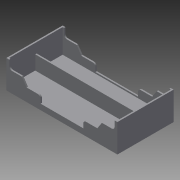
# Autodesk Inventor part: Badrepack
Saved by Autodesk Inventor 2015 (Build 190159000, 159)
## iProperties
Created: 2019-01-15
Part Number: Badrepack
Material: Типовые
Document SubType Name: Modeling
Designer: kostya
Density: 1 g/cm^3
Appearance: По умолчанию
Author: kostya
Autodesk Inventor part; units mm, degrees
ref_plane "YZ Plane" through (0, 0, 0) normal (1, 0, 0) x (0, 1, 0)
ref_plane "XZ Plane" through (0, 0, 0) normal (0, 1, 0) x (-1, 0, 0)
ref_plane "XY Plane" through (0, 0, 0) normal (0, 0, 1) x (1, 0, 0)
sketch "Эскиз1" plane through (0, 0, 0) normal (0, 0, 1) x (1, 0, 0)
  line L0 (-39.5, -20) -> (39.5, -20)
  line L1 (39.5, -20) -> (39.5, 20)
  line L2 (39.5, 20) -> (-39.5, 20)
  line L3 (-39.5, 20) -> (-39.5, -20)
  line L4 (-39.5, -20) -> (39.5, 20) construction
  line L5 (39.5, -20) -> (-39.5, 20) construction
  line L6 (-38.5, 19) -> (38.5, 19)
  line L7 (38.5, 19) -> (38.5, -19)
  line L8 (38.5, -19) -> (-38.5, -19)
  line L9 (-38.5, -19) -> (-38.5, 19)
  point P0 (0, 0)
  dimension "d0" = 79
  dimension "d1" = 40
  dimension "d2" = 1
  constraints: 20 end point, 4 parallel, 2 midpoint, 2 perpendicular, 1 horizontal, 3 other
  measures "d0" distance of L2.end L1.end
  measures "d1" distance of L1.end L0.end
  measures "d2" distance between parallel lines of L2 L6
extrude "Выдавливание1" add sketch "Эскиз1" along normal blind 3 contours L6 L7 L8 L9
extrude "Выдавливание2" add sketch "Эскиз1" along normal blind 20
sketch "Эскиз2" plane through (-39.5, -20, 0) normal (0, -1, 0) x (1, 0, 0)
  line L0 (2, 20) -> (2, 16) construction
  line L1 (4, 14) -> (11, 14)
  arc A0 (2, 16) -> (4, 14) centre (4, 16) ccw
  line L2 (11, 14) -> (11, 9) construction
  line L3 (14.3166, 9) -> (22.3166, 9)
  line L4 (24.3166, 7) -> (24.3166, 4)
  arc A1 (24.3166, 7) -> (22.3166, 9) centre (22.3166, 7) ccw
  line L5 (24.3166, 4) -> (39.5, 4)
  line L6 (39.5, 0) -> (39.5, 20) construction
  line L7 (77, 20) -> (77, 16) construction
  line L8 (75, 14) -> (68, 14)
  arc A2 (75, 14) -> (77, 16) centre (75, 16) ccw
  line L9 (68, 14) -> (64.6834, 9)
  line L10 (64.6834, 9) -> (56.6834, 9)
  line L11 (54.6834, 7) -> (54.6834, 4)
  arc A3 (56.6834, 9) -> (54.6834, 7) centre (56.6834, 7) ccw
  line L12 (54.6834, 4) -> (39.5, 4)
  line L13 (77, 20) -> (77, 16) construction
  line L14 (77, 20) -> (77, 16)
  line L15 (2, 20) -> (77, 20)
  line L16 (14.3166, 9) -> (22.3166, 9)
  line L17 (24.3166, 7) -> (24.3166, 4)
  line L18 (24.3166, 4) -> (54.6834, 4)
  line L19 (54.6834, 4) -> (54.6834, 7)
  line L20 (56.6834, 9) -> (64.6834, 9)
  line L21 (64.6834, 9) -> (68, 14)
  line L22 (68, 14) -> (75, 14)
  line L23 (77, 16) -> (77, 20)
  line L24 (77, 20) -> (2, 20)
  line L25 (11, 14) -> (14.3166, 9)
  line L26 (2, 20) -> (2, 16)
  line L27 (0, 20) -> (79, 20) projected
  point P0 (24.3166, 9)
  dimension "d10" = 2
  dimension "d11" = 5
  dimension "d12" = 6
  dimension "d13" = 10
  dimension "d14" = 5
  dimension "d15" = 2
  constraints: 54 end point, 10 symmetric about line, 8 point on circle, 5 collinear, 4 centre point, 4 perpendicular, 4 tangent, 2 horizontal, 2 point on line, 2 vertical, 2 other
  measures "d10" radius of A0
  measures "d11" distance of L1.end L2.end
  measures "d12" distance of L1.end L3.start
  measures "d13" distance of L3.start point (24.317, 9)
  measures "d14" distance of point (24.317, 9) L4.end
  measures "d15" radius of A1
extrude "Выдавливание3" cut sketch "Эскиз2" against normal up to surface (40 mm away)
sketch "Эскиз3" plane through (0, 0, 3) normal (0, 0, 1) x (1, 0, 0)
  line L0 (38.5, 19) -> (-38.5, 19) projected
  line L1 (-38.5, 19) -> (-38.5, -19) projected
  line L2 (-38.5, -19) -> (38.5, -19) projected
  line L3 (38.5, -19) -> (38.5, 19) projected
  line L4 (-39.5, 20) -> (-39.5, -20) projected
  line L5 (39.5, 0.5) -> (-39.5, 0.5)
  line L6 (-39.5, 0.5) -> (-39.5, -0.5)
  line L7 (-39.5, -0.5) -> (39.5, -0.5)
  line L8 (39.5, -0.5) -> (39.5, 0.5)
  line L9 (39.5, 0.5) -> (-39.5, -0.5) construction
  line L10 (-39.5, 0.5) -> (39.5, -0.5) construction
  point P0 (0, 0)
  dimension "d18" = 1
  constraints: 12 end point, 2 midpoint, 2 parallel, 1 horizontal, 1 perpendicular, 1 point on line
  measures "d18" distance of L6.end L5.end
extrude "Выдавливание4" add sketch "Эскиз3" along normal blind 10 contours L5 L8 L7 L3 | L3 L7 L1 L5 | L1 L7 L4 L5
